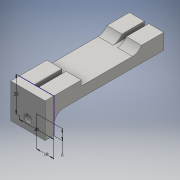
# Autodesk Inventor part: support_lcd
Saved by Autodesk Inventor 2016 (Build 200138000, 138)
## iProperties
Created: 2019-02-18
Part Number: support_lcd
Material: Generic
Document SubType Name: Modeling
Designer: mbouhier
Density: 1 g/cm^3
Appearance: Default
Author: mbouhier
Autodesk Inventor part; units mm, degrees
ref_plane "YZ Plane" through (0, 0, 0) normal (1, 0, 0) x (0, 1, 0)
ref_plane "XZ Plane" through (0, 0, 0) normal (0, 1, 0) x (-1, 0, 0)
ref_plane "XY Plane" through (0, 0, 0) normal (0, 0, 1) x (1, 0, 0)
sketch "Sketch1" plane through (0, 0, 0) normal (0, 1, 0) x (-1, 0, 0)
  line L0 (0, 0) -> (20, 0)
  line L1 (20, 0) -> (20, -20)
  line L2 (20, -20) -> (0, -20)
  line L3 (0, -20) -> (0, 0)
  point P0 (10, -14)
  dimension "d0" = 20
  dimension "d1" = 20
  dimension "d4" = 10
  dimension "d5" = 6
  constraints: 8 end point, 2 parallel, 1 horizontal, 1 perpendicular
  measures "d0" distance of L1.end L2.end
  measures "d1" distance of L0.end L1.end
  measures "d4" distance from line of point (10, -14) L3
  measures "d5" distance from line of L2 point (10, -14)
extrude "Extrusion1" add sketch "Sketch1" against normal blind 5
hole "Hole1" at (-10, 0, -14) direction (0, -1, 0) diameter 4.5 end through all counterbore diameter 8 counterbore depth 2
sketch "Sketch2" plane through (0, 0, 0) normal (0, 1, 0) x (1, 0, 0)
  line L0 (-20, 0) -> (-20, 20) projected
  line L1 (0, 20) -> (0, 0) projected
  line L2 (-20, 0) -> (0, 0)
  line L3 (0, 0) -> (0, 9)
  line L4 (0, 9) -> (-20, 9)
  line L5 (-20, 9) -> (-20, 0)
  line L6 (-20, 3) -> (0, 3) construction
  dimension "d13" = 9
  dimension "d14" = 3
  constraints: 10 end point, 3 point on line, 2 parallel, 2 perpendicular, 1 horizontal
  measures "d13" distance of L3.end L2.end
  measures "d14" distance between parallel lines of L6 L2
extrude "Extrusion2" add sketch "Sketch2" along normal blind 64
sketch "Sketch3" plane through (0, 64, 0) normal (0, 1, 0) x (1, 0, 0)
  line L0 (-11.25, 0) -> (-8.75, 0)
  line L1 (-8.75, 0) -> (-8.75, 3)
  line L2 (-8.75, 3) -> (-11.25, 3)
  line L3 (-11.25, 3) -> (-11.25, 0)
  line L4 (-20, 9) -> (-20, 0) projected
  point P0 (0, 0)
  dimension "d17" = 2.5
  dimension "d18" = 3
  dimension "d19" = 8.75
  constraints: 8 end point, 2 parallel, 1 horizontal, 1 perpendicular
  measures "d17" distance of L2.end L1.end
  measures "d18" distance of L1.end L0.end
  measures "d19" distance between parallel lines of L3 L4
fillet "Fillet1" radius 6 1 edges at (-10, 0, -9)
extrude "Extrusion3" cut sketch "Sketch3" against normal blind 64
sketch "Sketch4" plane through (0, -5, -20) normal (1, 0, 0) x (0, 0, -1)
  line L0 (-20, 0) -> (-20, 69) projected
  line L1 (-17, 5) -> (-20, 5) projected
  line L2 (-20, 56) -> (-17, 56)
  line L3 (-17, 56) -> (-17, 21)
  line L4 (-17, 21) -> (-20, 21)
  line L5 (-20, 21) -> (-20, 56)
  line L6 (-20, 69) -> (-11, 69) projected
  dimension "d23" = 16
  dimension "d25" = 13
  constraints: 8 end point, 2 parallel, 2 point on line, 1 horizontal, 1 perpendicular
  measures "d23" distance from line of point (-20, 21) L1
  measures "d25" distance from line of L2.start L6
extrude "Extrusion4" cut sketch "Sketch4" against normal blind 64
fillet "Fillet2" radius 6 2 edges at (-15.625, 51, -3) (-4.375, 51, -3)
body "Solid1"
